Autodesk Inventor part; units mm, degrees
(part 2 of 2)
  spline S293 degree 2 poles (26.5996, -155.7502) (26.5996, -155.8896) (26.8686, -156.1038) (27.3069, -156.1336) knots 0 0 0 1 2 2 2
  line L144 (27.3069, -156.1336) -> (27.3069, -156.298)
  line L145 (27.3069, -156.298) -> (25.3844, -156.298)
  line L146 (25.3844, -156.298) -> (25.3844, -156.1336)
  spline S294 degree 2 poles (25.3844, -156.1336) (25.7679, -156.0639) (25.8775, -155.9593) knots 0 0 0 1 1 1
  spline S295 degree 2 poles (25.8775, -155.9593) (26.1066, -155.7402) (26.3855, -155.0778) knots 0 0 0 1 1 1
  line L147 (26.3855, -155.0778) -> (28.537, -150.0625)
  line L148 (28.537, -150.0625) -> (28.6964, -150.0625)
  line L149 (28.6964, -150.0625) -> (30.818, -155.1326)
  spline S296 degree 2 poles (30.818, -155.1326) (31.072, -155.7452) (31.4904, -156.1087) (31.8639, -156.1336) knots 0 0 0 1 2 2 2
  line L150 (31.8639, -156.1336) -> (31.8639, -156.298)
  line L151 (31.8639, -156.298) -> (29.4584, -156.298)
  line L152 (29.4584, -156.298) -> (29.4584, -156.1336)
  spline S297 degree 2 poles (29.4584, -156.1336) (29.822, -156.1137) (30.0809, -155.9095) (30.0809, -155.7601) knots 0 0 0 1 2 2 2
  spline S298 degree 2 poles (30.0809, -155.7601) (30.0809, -155.5609) (29.9016, -155.1326) knots 0 0 0 1 1 1
  line L153 (29.9016, -155.1326) -> (29.5381, -154.261)
  line L154 (29.3986, -153.9273) -> (28.3727, -151.462)
  line L155 (28.3727, -151.462) -> (27.3069, -153.9273)
  line L156 (27.3069, -153.9273) -> (29.3986, -153.9273)
  line L157 (35.8632, -152.1792) -> (35.8632, -154.6794)
  spline S299 degree 2 poles (35.8632, -154.6794) (35.8632, -155.3866) (35.9329, -155.7053) (36.0773, -155.8298) (36.1769, -155.8298) knots 0 0 0 1 2 3 3 3
  spline S300 degree 2 poles (36.1769, -155.8298) (36.3164, -155.8298) (36.4907, -155.7551) knots 0 0 0 1 1 1
  line L158 (36.4907, -155.7551) -> (36.5554, -155.9195)
  line L159 (36.5554, -155.9195) -> (35.3253, -156.4225)
  line L160 (35.3253, -156.4225) -> (35.1211, -156.4225)
  line L161 (35.1211, -156.4225) -> (35.1211, -155.5509)
  spline S301 degree 2 poles (35.1211, -155.5509) (34.5882, -156.1237) (34.0354, -156.4225) (33.7216, -156.4225) knots 0 0 0 1 2 2 2
  spline S302 degree 2 poles (33.7216, -156.4225) (33.378, -156.4225) (32.87, -156.0241) (32.6707, -155.3916) (32.6707, -154.8188) knots 0 0 0 1 2 3 3 3
  line L162 (32.6707, -154.8188) -> (32.6707, -152.9811)
  spline S303 degree 2 poles (32.6707, -152.9811) (32.6707, -152.6872) (32.5462, -152.4631) (32.2972, -152.3386) (31.9735, -152.3436) knots 0 0 0 1 2 3 3 3
  line L163 (31.9735, -152.3436) -> (31.9735, -152.1792)
  line L164 (31.9735, -152.1792) -> (33.4178, -152.1792)
  line L165 (33.4178, -152.1792) -> (33.4178, -154.9334)
  spline S304 degree 2 poles (33.4178, -154.9334) (33.4178, -155.5111) (33.8162, -155.8697) (34.1001, -155.8697) knots 0 0 0 1 2 2 2
  spline S305 degree 2 poles (34.1001, -155.8697) (34.2943, -155.8697) (34.7824, -155.6256) (35.1211, -155.287) knots 0 0 0 1 2 2 2
  line L166 (35.1211, -155.287) -> (35.1211, -152.9512)
  spline S306 degree 2 poles (35.1211, -152.9512) (35.1211, -152.6025) (34.8621, -152.3535) (34.4537, -152.3436) knots 0 0 0 1 2 2 2
  line L167 (34.4537, -152.3436) -> (34.4537, -152.1792)
  line L168 (34.4537, -152.1792) -> (35.8632, -152.1792)
  spline S307 degree 2 poles (37.9599, -154.7939) (37.5814, -154.6096) (37.178, -153.9522) (37.178, -153.5488) knots 0 0 0 1 2 2 2
  spline S308 degree 2 poles (37.178, -153.5488) (37.178, -152.9412) (38.0994, -152.0597) (38.8215, -152.0597) knots 0 0 0 1 2 2 2
  spline S309 degree 2 poles (38.8215, -152.0597) (39.4092, -152.0597) (39.8425, -152.3485) knots 0 0 0 1 1 1
  line L169 (39.8425, -152.3485) -> (40.7141, -152.3485)
  spline S310 degree 2 poles (40.7141, -152.3485) (40.9083, -152.3485) (40.9731, -152.3685) (40.988, -152.3983) knots 0 0 0 1 2 2 2
  spline S311 degree 2 poles (40.988, -152.3983) (41.0129, -152.4382) (41.0129, -152.5428) knots 0 0 0 1 1 1
  spline S312 degree 2 poles (41.0129, -152.5428) (41.0129, -152.6573) (40.988, -152.7022) knots 0 0 0 1 1 1
  spline S313 degree 2 poles (40.988, -152.7022) (40.978, -152.7271) (40.9083, -152.752) (40.7141, -152.752) knots 0 0 0 1 2 2 2
  line L170 (40.7141, -152.752) -> (40.1762, -152.752)
  spline S314 degree 2 poles (40.1762, -152.752) (40.4302, -153.0757) (40.4302, -153.5787) knots 0 0 0 1 1 1
  spline S315 degree 2 poles (40.4302, -153.5787) (40.4302, -154.1564) (39.5487, -154.9732) (38.8066, -154.9732) knots 0 0 0 1 2 2 2
  spline S316 degree 2 poles (38.8066, -154.9732) (38.5028, -154.9732) (38.1791, -154.8836) knots 0 0 0 1 1 1
  spline S317 degree 2 poles (38.1791, -154.8836) (37.9848, -155.0529) (37.8454, -155.3069) (37.8454, -155.3965) knots 0 0 0 1 2 2 2
  spline S318 degree 2 poles (37.8454, -155.3965) (37.8454, -155.4762) (37.9948, -155.6207) (38.2089, -155.6505) knots 0 0 0 1 2 2 2
  spline S319 degree 2 poles (38.2089, -155.6505) (38.3334, -155.6705) (38.8414, -155.6804) knots 0 0 0 1 1 1
  spline S320 degree 2 poles (38.8414, -155.6804) (39.7678, -155.7053) (40.0417, -155.7452) knots 0 0 0 1 1 1
  spline S321 degree 2 poles (40.0417, -155.7452) (40.4601, -155.8049) (40.9581, -156.308) (40.9581, -156.6715) knots 0 0 0 1 2 2 2
  spline S322 degree 2 poles (40.9581, -156.6715) (40.9581, -157.1795) (40.48, -157.6228) knots 0 0 0 1 1 1
  spline S323 degree 2 poles (40.48, -157.6228) (39.7778, -158.2802) (38.6472, -158.2802) knots 0 0 0 1 1 1
  spline S324 degree 2 poles (38.6472, -158.2802) (37.7806, -158.2802) (37.183, -157.8917) knots 0 0 0 1 1 1
  spline S325 degree 2 poles (37.183, -157.8917) (36.8443, -157.6676) (36.8443, -157.4236) knots 0 0 0 1 1 1
  spline S326 degree 2 poles (36.8443, -157.4236) (36.8443, -157.314) (36.8941, -157.2094) knots 0 0 0 1 1 1
  spline S327 degree 2 poles (36.8941, -157.2094) (36.9688, -157.0401) (37.2079, -156.7462) knots 0 0 0 1 1 1
  spline S328 degree 2 poles (37.2079, -156.7462) (37.2427, -156.7064) (37.6661, -156.2631) knots 0 0 0 1 1 1
  spline S329 degree 2 poles (37.6661, -156.2631) (37.437, -156.1237) (37.2427, -155.8996) (37.2427, -155.7601) knots 0 0 0 1 2 2 2
  spline S330 degree 2 poles (37.2427, -155.7601) (37.2427, -155.6057) (37.4967, -155.1824) (37.9599, -154.7939) knots 0 0 0 1 2 2 2
  spline S331 degree 2 poles (37.9151, -156.298) (37.7009, -156.5271) (37.4868, -156.9205) (37.4868, -157.0849) knots 0 0 0 1 2 2 2
  spline S332 degree 2 poles (37.4868, -157.0849) (37.4868, -157.2991) (37.7458, -157.4584) knots 0 0 0 1 1 1
  spline S333 degree 2 poles (37.7458, -157.4584) (38.199, -157.7373) (39.0506, -157.7373) knots 0 0 0 1 1 1
  spline S334 degree 2 poles (39.0506, -157.7373) (39.8574, -157.7373) (40.6294, -157.1696) (40.6294, -156.8508) knots 0 0 0 1 2 2 2
  spline S335 degree 2 poles (40.6294, -156.8508) (40.6294, -156.6167) (40.4003, -156.5171) knots 0 0 0 1 1 1
  spline S336 degree 2 poles (40.4003, -156.5171) (40.1662, -156.4225) (39.474, -156.4026) knots 0 0 0 1 1 1
  spline S337 degree 2 poles (39.474, -156.4026) (38.458, -156.3777) (37.9151, -156.298) knots 0 0 0 1 1 1
  spline S338 degree 2 poles (38.7418, -152.2738) (38.4081, -152.2738) (37.9599, -152.8018) (37.9599, -153.3496) knots 0 0 0 1 2 2 2
  spline S339 degree 2 poles (37.9599, -153.3496) (37.9599, -154.0618) (38.2637, -154.4503) knots 0 0 0 1 1 1
  spline S340 degree 2 poles (38.2637, -154.4503) (38.4978, -154.7491) (38.8614, -154.7491) knots 0 0 0 1 1 1
  spline S341 degree 2 poles (38.8614, -154.7491) (39.2, -154.7491) (39.6433, -154.2361) (39.6433, -153.6883) knots 0 0 0 1 2 2 2
  spline S342 degree 2 poles (39.6433, -153.6883) (39.6433, -152.9761) (39.3345, -152.5727) knots 0 0 0 1 1 1
  spline S343 degree 2 poles (39.3345, -152.5727) (39.1054, -152.2738) (38.7418, -152.2738) knots 0 0 0 1 1 1
  line L171 (47.7016, -155.1276) -> (47.2732, -156.298)
  line L172 (47.2732, -156.298) -> (43.6774, -156.298)
  line L173 (43.6774, -156.298) -> (43.6774, -156.1336)
  spline S344 degree 2 poles (43.6774, -156.1336) (45.2661, -154.6843) (46.5611, -152.8516) (46.5611, -152.0896) knots 0 0 0 1 2 2 2
  spline S345 degree 2 poles (46.5611, -152.0896) (46.5611, -151.5118) (45.8489, -150.7648) (45.3558, -150.7648) knots 0 0 0 1 2 2 2
  spline S346 degree 2 poles (45.3558, -150.7648) (44.9026, -150.7648) (44.1904, -151.2927) (44.0161, -151.8007) knots 0 0 0 1 2 2 2
  line L174 (44.0161, -151.8007) -> (43.8517, -151.8007)
  spline S347 degree 2 poles (43.8517, -151.8007) (43.9663, -150.969) (44.8926, -150.0775) (45.5899, -150.0775) knots 0 0 0 1 2 2 2
  spline S348 degree 2 poles (45.5899, -150.0775) (46.332, -150.0775) (47.328, -151.0287) (47.328, -151.6762) knots 0 0 0 1 2 2 2
  spline S349 degree 2 poles (47.328, -151.6762) (47.328, -152.1394) (47.1139, -152.6025) knots 0 0 0 1 1 1
  spline S350 degree 2 poles (47.1139, -152.6025) (46.7802, -153.3297) (46.0331, -154.1465) knots 0 0 0 1 1 1
  spline S351 degree 2 poles (46.0331, -154.1465) (44.9125, -155.3667) (44.6336, -155.6207) knots 0 0 0 1 1 1
  line L175 (44.6336, -155.6207) -> (46.2274, -155.6207)
  spline S352 degree 2 poles (46.2274, -155.6207) (46.7154, -155.6207) (47.1039, -155.5509) (47.4177, -155.3268) (47.5372, -155.1276) knots 0 0 0 1 2 3 3 3
  line L176 (47.5372, -155.1276) -> (47.7016, -155.1276)
  line L177 (49.0114, -150.202) -> (52.2785, -150.202)
  line L178 (52.2785, -150.202) -> (52.2785, -150.3713)
  line L179 (52.2785, -150.3713) -> (50.2465, -156.4225)
  line L180 (50.2465, -156.4225) -> (49.7435, -156.4225)
  line L181 (49.7435, -156.4225) -> (51.5663, -150.9341)
  line L182 (51.5663, -150.9341) -> (49.888, -150.9341)
  spline S353 degree 2 poles (49.888, -150.9341) (49.38, -150.9341) (49.1658, -151.0536) knots 0 0 0 1 1 1
  spline S354 degree 2 poles (49.1658, -151.0536) (48.7873, -151.2628) (48.5582, -151.6961) knots 0 0 0 1 1 1
  line L183 (48.5582, -151.6961) -> (48.4287, -151.6463)
  line L184 (48.4287, -151.6463) -> (49.0114, -150.202)
  line L185 (54.1811, -150.8245) -> (54.1811, -152.1792)
  line L186 (54.1811, -152.1792) -> (55.1423, -152.1792)
  line L187 (55.1423, -152.1792) -> (55.1423, -152.493)
  line L188 (55.1423, -152.493) -> (54.1811, -152.493)
  line L189 (54.1811, -152.493) -> (54.1811, -155.1674)
  spline S355 degree 2 poles (54.1811, -155.1674) (54.1811, -155.5659) (54.4101, -155.8448) (54.5894, -155.8448) knots 0 0 0 1 2 2 2
  spline S356 degree 2 poles (54.5894, -155.8448) (54.7389, -155.8448) (55.0227, -155.6605) (55.0974, -155.4812) knots 0 0 0 1 2 2 2
  line L190 (55.0974, -155.4812) -> (55.2718, -155.4812)
  spline S357 degree 2 poles (55.2718, -155.4812) (55.1124, -155.9245) (54.5347, -156.3677) (54.2309, -156.3677) knots 0 0 0 1 2 2 2
  spline S358 degree 2 poles (54.2309, -156.3677) (54.0217, -156.3677) (53.6232, -156.1386) (53.434, -155.7103) (53.434, -155.2671) knots 0 0 0 1 2 3 3 3
  line L191 (53.434, -155.2671) -> (53.434, -152.493)
  line L192 (53.434, -152.493) -> (52.7816, -152.493)
  line L193 (52.7816, -152.493) -> (52.7816, -152.3436)
  spline S359 degree 2 poles (52.7816, -152.3436) (53.0306, -152.244) (53.5485, -151.7758) (53.7527, -151.4521) knots 0 0 0 1 2 2 2
  spline S360 degree 2 poles (53.7527, -151.4521) (53.8573, -151.2778) (54.0416, -150.8245) knots 0 0 0 1 1 1
  line L194 (54.0416, -150.8245) -> (54.1811, -150.8245)
  line L195 (56.7509, -149.9032) -> (56.7509, -152.9163)
  spline S361 degree 2 poles (56.7509, -152.9163) (57.249, -152.3685) (57.8317, -152.0597) (58.1255, -152.0597) knots 0 0 0 1 2 2 2
  spline S362 degree 2 poles (58.1255, -152.0597) (58.4741, -152.0597) (58.9821, -152.4482) (59.1017, -152.8615) knots 0 0 0 1 2 2 2
  spline S363 degree 2 poles (59.1017, -152.8615) (59.1863, -153.1454) (59.1863, -153.9124) knots 0 0 0 1 1 1
  line L196 (59.1863, -153.9124) -> (59.1863, -155.3667)
  spline S364 degree 2 poles (59.1863, -155.3667) (59.1863, -155.7551) (59.2511, -155.8996) knots 0 0 0 1 1 1
  spline S365 degree 2 poles (59.2511, -155.8996) (59.2959, -156.0091) (59.5101, -156.1336) (59.7989, -156.1336) knots 0 0 0 1 2 2 2
  line L197 (59.7989, -156.1336) -> (59.7989, -156.298)
  line L198 (59.7989, -156.298) -> (57.7719, -156.298)
  line L199 (57.7719, -156.298) -> (57.7719, -156.1336)
  line L200 (57.7719, -156.1336) -> (57.8665, -156.1336)
  spline S366 degree 2 poles (57.8665, -156.1336) (58.1554, -156.1336) (58.3795, -155.9593) (58.4243, -155.79) knots 0 0 0 1 2 2 2
  spline S367 degree 2 poles (58.4243, -155.79) (58.4393, -155.7153) (58.4393, -155.3667) knots 0 0 0 1 1 1
  line L201 (58.4393, -155.3667) -> (58.4393, -153.9124)
  spline S368 degree 2 poles (58.4393, -153.9124) (58.4393, -153.2351) (58.2998, -152.8117) (57.996, -152.6025) (57.7769, -152.6025) knots 0 0 0 1 2 3 3 3
  spline S369 degree 2 poles (57.7769, -152.6025) (57.5578, -152.6025) (57.0846, -152.8366) (56.7509, -153.1902) knots 0 0 0 1 2 2 2
  line L202 (56.7509, -153.1902) -> (56.7509, -155.3667)
  spline S370 degree 2 poles (56.7509, -155.3667) (56.7509, -155.79) (56.8456, -155.9942) (57.1045, -156.1336) (57.4183, -156.1336) knots 0 0 0 1 2 3 3 3
  line L203 (57.4183, -156.1336) -> (57.4183, -156.298)
  line L204 (57.4183, -156.298) -> (55.3763, -156.298)
  line L205 (55.3763, -156.298) -> (55.3763, -156.1336)
  spline S371 degree 2 poles (55.3763, -156.1336) (55.6503, -156.1336) (55.8047, -156.049) knots 0 0 0 1 1 1
  spline S372 degree 2 poles (55.8047, -156.049) (55.8943, -156.0042) (56.0039, -155.7502) (56.0039, -155.3667) knots 0 0 0 1 2 2 2
  line L206 (56.0039, -155.3667) -> (56.0039, -151.6363)
  spline S373 degree 2 poles (56.0039, -151.6363) (56.0039, -150.9341) (55.9341, -150.6154) (55.7947, -150.5008) (55.6801, -150.5008) knots 0 0 0 1 2 3 3 3
  spline S374 degree 2 poles (55.6801, -150.5008) (55.5855, -150.5008) (55.3763, -150.5705) knots 0 0 0 1 1 1
  line L207 (55.3763, -150.5705) -> (55.3116, -150.4062)
  line L208 (55.3116, -150.4062) -> (56.5418, -149.9032)
  line L209 (56.5418, -149.9032) -> (56.7509, -149.9032)
  line L210 (66.383, -155.1276) -> (65.9547, -156.298)
  line L211 (65.9547, -156.298) -> (62.3589, -156.298)
  line L212 (62.3589, -156.298) -> (62.3589, -156.1336)
  spline S375 degree 2 poles (62.3589, -156.1336) (63.9476, -154.6843) (65.2425, -152.8516) (65.2425, -152.0896) knots 0 0 0 1 2 2 2
  spline S376 degree 2 poles (65.2425, -152.0896) (65.2425, -151.5118) (64.5303, -150.7648) (64.0372, -150.7648) knots 0 0 0 1 2 2 2
  spline S377 degree 2 poles (64.0372, -150.7648) (63.584, -150.7648) (62.8718, -151.2927) (62.6975, -151.8007) knots 0 0 0 1 2 2 2
  line L213 (62.6975, -151.8007) -> (62.5332, -151.8007)
  spline S378 degree 2 poles (62.5332, -151.8007) (62.6477, -150.969) (63.5741, -150.0775) (64.2713, -150.0775) knots 0 0 0 1 2 2 2
  spline S379 degree 2 poles (64.2713, -150.0775) (65.0134, -150.0775) (66.0095, -151.0287) (66.0095, -151.6762) knots 0 0 0 1 2 2 2
  spline S380 degree 2 poles (66.0095, -151.6762) (66.0095, -152.1394) (65.7953, -152.6025) knots 0 0 0 1 1 1
  spline S381 degree 2 poles (65.7953, -152.6025) (65.4616, -153.3297) (64.7146, -154.1465) knots 0 0 0 1 1 1
  spline S382 degree 2 poles (64.7146, -154.1465) (63.594, -155.3667) (63.3151, -155.6207) knots 0 0 0 1 1 1
  line L214 (63.3151, -155.6207) -> (64.9088, -155.6207)
  spline S383 degree 2 poles (64.9088, -155.6207) (65.3969, -155.6207) (65.7854, -155.5509) (66.0991, -155.3268) (66.2187, -155.1276) knots 0 0 0 1 2 3 3 3
  line L215 (66.2187, -155.1276) -> (66.383, -155.1276)
  spline S384 degree 2 poles (67.1002, -153.2849) (67.1002, -152.244) (67.7277, -150.7399) (68.2507, -150.3713) knots 0 0 0 1 2 2 2
  spline S385 degree 2 poles (68.2507, -150.3713) (68.6541, -150.0775) (69.0874, -150.0775) knots 0 0 0 1 1 1
  spline S386 degree 2 poles (69.0874, -150.0775) (69.7896, -150.0775) (70.3474, -150.7897) knots 0 0 0 1 1 1
  spline S387 degree 2 poles (70.3474, -150.7897) (71.0447, -151.6762) (71.0447, -153.1902) knots 0 0 0 1 1 1
  spline S388 degree 2 poles (71.0447, -153.1902) (71.0447, -154.2511) (70.4321, -155.7352) (69.4858, -156.4026) (69.0425, -156.4026) knots 0 0 0 1 2 3 3 3
  spline S389 degree 2 poles (69.0425, -156.4026) (68.171, -156.4026) (67.5883, -155.3716) knots 0 0 0 1 1 1
  spline S390 degree 2 poles (67.5883, -155.3716) (67.1002, -154.5051) (67.1002, -153.2849) knots 0 0 0 1 1 1
  spline S391 degree 2 poles (67.9817, -153.3994) (67.9817, -154.6545) (68.2905, -155.4513) knots 0 0 0 1 1 1
  spline S392 degree 2 poles (68.2905, -155.4513) (68.5495, -156.1187) (69.0575, -156.1187) knots 0 0 0 1 1 1
  spline S393 degree 2 poles (69.0575, -156.1187) (69.3015, -156.1187) (69.8195, -155.6854) (69.954, -155.1724) knots 0 0 0 1 2 2 2
  spline S394 degree 2 poles (69.954, -155.1724) (70.1631, -154.4005) (70.1631, -152.996) knots 0 0 0 1 1 1
  spline S395 degree 2 poles (70.1631, -152.996) (70.1631, -151.9501) (69.949, -151.2578) knots 0 0 0 1 1 1
  spline S396 degree 2 poles (69.949, -151.2578) (69.7846, -150.7399) (69.5306, -150.5257) knots 0 0 0 1 1 1
  spline S397 degree 2 poles (69.5306, -150.5257) (69.3463, -150.3763) (69.0824, -150.3763) knots 0 0 0 1 1 1
  spline S398 degree 2 poles (69.0824, -150.3763) (68.7786, -150.3763) (68.5395, -150.6502) knots 0 0 0 1 1 1
  spline S399 degree 2 poles (68.5395, -150.6502) (68.2158, -151.0238) (67.9817, -152.6225) (67.9817, -153.3994) knots 0 0 0 1 2 2 2
  line L216 (75.5967, -155.1276) -> (75.1684, -156.298)
  line L217 (75.1684, -156.298) -> (71.5726, -156.298)
  line L218 (71.5726, -156.298) -> (71.5726, -156.1336)
  spline S400 degree 2 poles (71.5726, -156.1336) (73.1613, -154.6843) (74.4562, -152.8516) (74.4562, -152.0896) knots 0 0 0 1 2 2 2
  spline S401 degree 2 poles (74.4562, -152.0896) (74.4562, -151.5118) (73.744, -150.7648) (73.251, -150.7648) knots 0 0 0 1 2 2 2
  spline S402 degree 2 poles (73.251, -150.7648) (72.7978, -150.7648) (72.0856, -151.2927) (71.9112, -151.8007) knots 0 0 0 1 2 2 2
  line L219 (71.9112, -151.8007) -> (71.7469, -151.8007)
  spline S403 degree 2 poles (71.7469, -151.8007) (71.8614, -150.969) (72.7878, -150.0775) (73.4851, -150.0775) knots 0 0 0 1 2 2 2
  spline S404 degree 2 poles (73.4851, -150.0775) (74.2271, -150.0775) (75.2232, -151.0287) (75.2232, -151.6762) knots 0 0 0 1 2 2 2
  spline S405 degree 2 poles (75.2232, -151.6762) (75.2232, -152.1394) (75.0091, -152.6025) knots 0 0 0 1 1 1
  spline S406 degree 2 poles (75.0091, -152.6025) (74.6754, -153.3297) (73.9283, -154.1465) knots 0 0 0 1 1 1
  spline S407 degree 2 poles (73.9283, -154.1465) (72.8077, -155.3667) (72.5288, -155.6207) knots 0 0 0 1 1 1
  line L220 (72.5288, -155.6207) -> (74.1225, -155.6207)
  spline S408 degree 2 poles (74.1225, -155.6207) (74.6106, -155.6207) (74.9991, -155.5509) (75.3129, -155.3268) (75.4324, -155.1276) knots 0 0 0 1 2 3 3 3
  line L221 (75.4324, -155.1276) -> (75.5967, -155.1276)
  line L222 (79.9795, -150.202) -> (79.6309, -150.964)
  line L223 (79.6309, -150.964) -> (77.7981, -150.964)
  line L224 (77.7981, -150.964) -> (77.3947, -151.7808)
  spline S409 degree 2 poles (77.3947, -151.7808) (78.585, -151.9551) (79.2822, -152.6673) knots 0 0 0 1 1 1
  spline S410 degree 2 poles (79.2822, -152.6673) (79.8799, -153.2799) (79.8799, -154.1066) knots 0 0 0 1 1 1
  spline S411 degree 2 poles (79.8799, -154.1066) (79.8799, -154.5847) (79.4864, -155.4065) (78.8938, -155.9792) (78.5302, -156.1536) knots 0 0 0 1 2 3 3 3
  spline S412 degree 2 poles (78.5302, -156.1536) (78.0122, -156.4026) (77.4694, -156.4026) knots 0 0 0 1 1 1
  spline S413 degree 2 poles (77.4694, -156.4026) (76.9165, -156.4026) (76.4185, -156.0291) (76.4185, -155.8049) knots 0 0 0 1 2 2 2
  spline S414 degree 2 poles (76.4185, -155.8049) (76.4185, -155.6804) (76.6227, -155.4862) (76.7821, -155.4862) knots 0 0 0 1 2 2 2
  spline S415 degree 2 poles (76.7821, -155.4862) (76.8966, -155.4862) (77.0759, -155.5609) (77.2851, -155.7103) knots 0 0 0 1 2 2 2
  spline S416 degree 2 poles (77.2851, -155.7103) (77.6238, -155.9394) (77.9724, -155.9444) knots 0 0 0 1 1 1
  spline S417 degree 2 poles (77.9724, -155.9444) (78.4953, -155.9444) (79.2972, -155.1475) (79.2972, -154.5748) knots 0 0 0 1 2 2 2
  spline S418 degree 2 poles (79.2972, -154.5748) (79.2972, -154.022) (78.585, -153.0607) (77.9574, -152.8018) knots 0 0 0 1 2 2 2
  spline S419 degree 2 poles (77.9574, -152.8018) (77.4694, -152.5976) (76.6227, -152.5677) knots 0 0 0 1 1 1
  line L225 (76.6227, -152.5677) -> (77.7931, -150.202)
  line L226 (77.7931, -150.202) -> (79.9795, -150.202)
  point P0 (106.8994, -178.9)
  dimension "d0" = 178.9
  constraints: 2 other
emboss "Emboss1" sketch "Sketch18" operation cut depth 1.5 direction (1, 0, 0)
body "Solid1"
